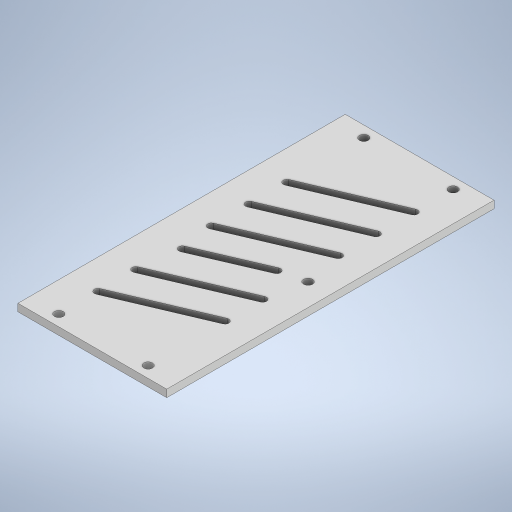
# Autodesk Inventor part: left_side
Saved by Autodesk Inventor 2024 (Build 280153000, 153)
## iProperties
Created: 2026-03-15
Part Number: left_side
Material: Generic
Document SubType Name: Modeling
Designer: HP
Density: 1 g/cm^3
Appearance: Default
Author: HP
Autodesk Inventor part; units mm, degrees
ref_plane "YZ Plane" through (0, 0, 0) normal (1, 0, 0) x (0, 1, 0)
ref_plane "XZ Plane" through (0, 0, 0) normal (0, 1, 0) x (-1, 0, 0)
ref_plane "XY Plane" through (0, 0, 0) normal (0, 0, 1) x (1, 0, 0)
sketch "Sketch1" plane through (0, 0, 0) normal (0, 1, 0) x (-1, 0, 0)
  line L0 (0, 0) -> (0, 110)
  line L1 (0, 110) -> (50, 110)
  line L2 (50, 110) -> (50, -110)
  line L3 (50, -110) -> (0, -110)
  line L4 (0, -110) -> (0, 0)
  line L5 (50, 0) -> (0, 0)
  line L6 (50, 110) -> (50, 102.5)
  line L7 (50, 102.5) -> (30, 102.5)
  line L8 (0, 110) -> (-50, 110)
  line L9 (-50, 110) -> (-50, -110)
  line L10 (-50, -110) -> (0, -110)
  circle A0 centre (30, 102.5) radius 3
  line L11 (30, 102.5) -> (-30, 102.5)
  circle A1 centre (-30, 102.5) radius 3
  circle A2 centre (30, -102.5) radius 3
  circle A3 centre (-30, -102.5) radius 3
  line L12 (30, 102.5) -> (30, -102.5)
  line L13 (-30, 102.5) -> (-30, -102.5)
  line L14 (30, 76.2) -> (-30, 50.8) construction
  line L15 (29.0254, 78.5022) -> (-30.9746, 53.1022)
  line L16 (-29.0254, 48.4978) -> (30.9746, 73.8978)
  arc A4 (30.9746, 73.8978) -> (29.0254, 78.5022) centre (30, 76.2) ccw
  arc A5 (-30.9746, 53.1022) -> (-29.0254, 48.4978) centre (-30, 50.8) ccw
  line L17 (30, 50.8) -> (-30, 25.4) construction
  line L18 (29.0254, 53.1022) -> (-30.9746, 27.7022)
  line L19 (-29.0254, 23.0978) -> (30.9746, 48.4978)
  arc A6 (30.9746, 48.4978) -> (29.0254, 53.1022) centre (30, 50.8) ccw
  arc A7 (-30.9746, 27.7022) -> (-29.0254, 23.0978) centre (-30, 25.4) ccw
  line L20 (30, 25.4) -> (-30, 0) construction
  line L21 (29.0254, 27.7022) -> (-30.9746, 2.3022)
  line L22 (-29.0254, -2.3022) -> (30.9746, 23.0978)
  arc A8 (30.9746, 23.0978) -> (29.0254, 27.7022) centre (30, 25.4) ccw
  arc A9 (-30.9746, 2.3022) -> (-29.0254, -2.3022) centre (-30, 0) ccw
  line L23 (30, 0) -> (-30, -25.4) construction
  line L24 (29.0254, 2.3022) -> (-30.9746, -23.0978)
  line L25 (-29.0254, -27.7022) -> (30.9746, -2.3022)
  arc A10 (30.9746, -2.3022) -> (29.0254, 2.3022) centre (30, 0) ccw
  arc A11 (-30.9746, -23.0978) -> (-29.0254, -27.7022) centre (-30, -25.4) ccw
  line L26 (30, -25.4) -> (-30, -50.8) construction
  line L27 (29.0254, -23.0978) -> (-30.9746, -48.4978)
  line L28 (-29.0254, -53.1022) -> (30.9746, -27.7022)
  arc A12 (30.9746, -27.7022) -> (29.0254, -23.0978) centre (30, -25.4) ccw
  arc A13 (-30.9746, -48.4978) -> (-29.0254, -53.1022) centre (-30, -50.8) ccw
  line L29 (30, -50.8) -> (-30, -76.2) construction
  line L30 (29.0254, -48.4978) -> (-30.9746, -73.8978)
  line L31 (-29.0254, -78.5022) -> (30.9746, -53.1022)
  arc A14 (30.9746, -53.1022) -> (29.0254, -48.4978) centre (30, -50.8) ccw
  arc A15 (-30.9746, -73.8978) -> (-29.0254, -78.5022) centre (-30, -76.2) ccw
  point P0 (0, 63.5)
  point P1 (0, 38.1)
  point P2 (0, 12.7)
  point P3 (0, -12.7)
  point P4 (0, -38.1)
  point P5 (0, -63.5)
  dimension "d0" = 110
  dimension "d1" = 50
  dimension "d2" = 220
  dimension "d3" = 7.5
  dimension "d4" = 20
  dimension "d5" = 50
  dimension "d6" = 6
  dimension "d7" = 60
  dimension "d8" = 6
  dimension "d9" = 5
  dimension "d10" = 5
  dimension "d11" = 5
  dimension "d12" = 5
  dimension "d13" = 5
  dimension "d14" = 5
  constraints: 76 end point, 24 point on circle, 24 tangent, 16 centre point, 11 point on line, 10 parallel, 9 midpoint, 6 perpendicular, 3 horizontal, 2 coincident, 2 symmetric about line, 1 vertical, 2 other
  measures "d0" distance of L0.start L0.end
  measures "d1" distance of L0.end L1.end
  measures "d2" distance of L1.end L2.end
  measures "d3" distance of L1.end L6.end
  measures "d4" distance of L6.end L7.end
  measures "d5" distance of L0.end L8.end
  measures "d6" diameter of A0
  measures "d7" distance of L11.start L11.end
  measures "d8" diameter of A1
  measures "d9" diameter of A5
  measures "d10" diameter of A7
  measures "d11" diameter of A9
  measures "d12" diameter of A11
  measures "d13" diameter of A13
  measures "d14" diameter of A15
extrude "Extrusion1" add sketch "Sketch1" along normal blind 5 contours L4 L24 L13 A9 L22 L0 | L5 L24 L4 | L0 L22 L12 A10 L24 L5 | L21 L13 A7 L19 L0 | L0 L19 L12 A8 L21 | L22 A8 L12 L19 A6 L16 A4 A0 L7 L2 L5 A10 | L25 L12 A12 L27 L4 | L4 L27 L13 A11 L25 | L24 A11 L13 L27 A13 L30 A15 L31 L4 L10 L9 L8 L0 L11 A1 L15 A5 L18 A7 L21 A9 | L25 A10 L5 L2 L3 L4 L31 A14 L12 L28 A12 | L18 L13 A5 L16 L0 | L0 L16 L12 A6 L18 | L28 L12 A14 L30 L4 | L4 L30 L13 A13 L28 | L7 A0 L11 L0 L1 L2 | L15 L13 A1 L11 L0 | L0 L11 A0 L12 A4 L15
sketch "Sketch2" plane through (0, 5, 0) normal (0, 1, 0) x (1, 0, 0)
  line L0 (-30.9746, -23.0978) -> (29.0254, 2.3022) projected
  line L1 (29.0254, 2.3022) -> (-30.9746, -23.0978)
  line L2 (30.9746, -2.3022) -> (-29.0254, -27.7022) projected
  line L3 (30.9746, -2.3022) -> (-29.0254, -27.7022)
  arc A0 (30.9746, -2.3022) -> (29.0254, 2.3022) centre (30, 0) ccw projected
  arc A1 (30.9746, -2.3022) -> (29.0254, 2.3022) centre (30, 0) ccw
  arc A2 (-30.9746, -23.0978) -> (-29.0254, -27.7022) centre (-30, -25.4) ccw projected
  arc A3 (-30.9746, -23.0978) -> (-29.0254, -27.7022) centre (-30, -25.4) ccw
  point P0 (0, 0)
  constraints: 4 end point, 4 point on circle, 2 centre point, 2 collinear, 2 concentric
extrude "Extrusion2" add sketch "Sketch2" against normal blind 5
sketch "Sketch3" plane through (0, 5, 0) normal (0, 1, 0) x (1, 0, 0)
  line L0 (50, -110) -> (50, 110) projected
  line L1 (50, 110) -> (50, 0)
  line L2 (50, 0) -> (35, 0)
  circle A0 centre (35, 0) radius 3
  line L3 (-26.3927, -23.0836) -> (18.0573, -4.0336) construction
  line L4 (-25.4079, -25.3815) -> (19.0421, -6.3315)
  line L5 (17.0725, -1.7358) -> (-27.3775, -20.7858)
  arc A1 (-27.3775, -20.7858) -> (-25.4079, -25.3815) centre (-26.3927, -23.0836) ccw
  arc A2 (19.0421, -6.3315) -> (17.0725, -1.7358) centre (18.0573, -4.0336) ccw
  point P0 (0, 0)
  point P1 (-4.1677, -13.5586)
  dimension "d19" = 15
  dimension "d20" = 6
  dimension "d21" = 5
  constraints: 12 end point, 4 point on circle, 4 tangent, 3 centre point, 2 midpoint, 1 coincident, 1 horizontal, 1 parallel
  measures "d19" distance of L1.end L2.end
  measures "d20" diameter of A0
  measures "d21" diameter of A2
extrude "Extrusion3" cut sketch "Sketch3" against normal blind 5
body "Solid1"
